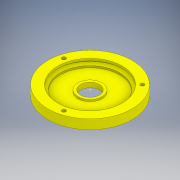
# Autodesk Inventor part: fix_plate_2
Saved by Autodesk Inventor 2018 (Build 220112000, 112)
## iProperties
Created: 2019-01-08
Part Number: fix_plate_2
Material: 一般
Document SubType Name: Modeling
Designer: lowyu
Density: 1 g/cm^3
Appearance: 既定
Author: lowyu
## iProperties of the stored document fix_plate_3D プリント.ipt
Created: 2019-01-08
Part Number: fix_plate_3D プリント
Material: 一般
Document SubType Name: Modeling
Designer: lowyu
Density: 1 g/cm^3
Appearance: 既定
Author: lowyu
Autodesk Inventor part; units mm, degrees
note: some values were not read from the file. Chosen so that the rebuilt part matches the saved one: second side of "押し出し6".
ref_plane "YZ Plane" through (0, 0, 0) normal (1, 0, 0) x (0, 1, 0)
ref_plane "XZ Plane" through (0, 0, 0) normal (0, 1, 0) x (-1, 0, 0)
ref_plane "XY Plane" through (0, 0, 0) normal (0, 0, 1) x (1, 0, 0)
sketch "スケッチ1" plane through (0, 0, 0) normal (0, 0, 1) x (1, 0, 0)
  circle A0 centre (0, 0) radius 46.9412
  dimension "d3" = 93.8824
  constraints: 1 centre point
  measures "d3" diameter of A0
extrude "押し出し1" add sketch "スケッチ1" along normal blind 10.5
sketch "スケッチ2" plane through (0, 0, 10.5) normal (0, 0, 1) x (1, 0, 0)
  circle A0 centre (0, 0) radius 46.9412
  arc A1 (35.7361, 3.8892) -> (3.8892, 35.7361) centre (0, 0) ccw
  circle A2 centre (29.2617, 29.2617) radius 2.1
  circle A3 centre (-39.9723, 10.7105) radius 2.1
  circle A4 centre (10.7105, -39.9723) radius 2.1
  circle A5 centre (0, 0) radius 35.9471
  dimension "d4" = 4.2
  constraints: 5 centre point, 2 point on circle, 1 coincident, 3 other
  measures "d4" diameter of A2
extrude "押し出し2" cut sketch "スケッチ2" against normal blind 5 contours A5 A1
sketch "スケッチ3" plane through (0, 0, 10.5) normal (0, 0, 1) x (1, 0, 0)
  circle A0 centre (0, 0) radius 46.9412
  arc A1 (-5.0225, 35.5945) -> (35.5945, -5.0225) centre (0, 0) ccw
  arc A2 (35.7361, 3.8892) -> (3.8892, 35.7361) centre (0, 0) ccw
  circle A3 centre (29.2617, 29.2617) radius 2.1
  circle A4 centre (-39.9723, 10.7105) radius 2.1
  circle A5 centre (10.7105, -39.9723) radius 2.1
  circle A6 centre (0, 0) radius 35.9471
  dimension "d7" = 4.2
  constraints: 6 centre point, 4 point on circle, 1 coincident, 3 other
  measures "d7" diameter of A3
extrude "押し出し3" cut sketch "スケッチ3" against normal blind 10.5 contours A3 | A4 | A5
sketch "スケッチ4" plane through (0, 0, 5.5) normal (0, 0, 1) x (1, 0, 0)
  circle A0 centre (0, 0) radius 10.5
  circle A1 centre (0, 0) radius 10.5
  constraints: 2 centre point
extrude "押し出し4" cut sketch "スケッチ4" against normal blind 10.5
sketch "スケッチ5" plane through (0, 0, 5.5) normal (0, 0, 1) x (1, 0, 0)
  circle A0 centre (0, 0) radius 10.5 projected
  circle A1 centre (0, 0) radius 35.9471 projected
  circle A2 centre (0, 0) radius 13.5
  circle A3 centre (0, 0) radius 32.9471
  dimension "d12" = 3
  dimension "d13" = 3
  constraints: 2 centre point, 2 coincident
  measures "d12" radial gap between concentric circles of A2 A0
  measures "d13" radial gap between concentric circles of A3 A1
extrude "押し出し5" cut sketch "スケッチ5" against normal blind 2 contours A3
sketch "スケッチ6" plane through (0, 0, 5.5) normal (0, 0, 1) x (1, 0, 0)
  point P0 (0, 0)
sketch "スケッチ7" plane through (0, 0, 5.5) normal (0, 0, 1) x (1, 0, 0)
  circle A0 centre (0, 0) radius 38.9471
  circle A1 centre (0, 0) radius 35.9471 projected
  dimension "d16" = 3
  constraints: 1 centre point, 1 coincident
  measures "d16" radial gap between concentric circles of A1 A0
extrude "押し出し6" cut sketch "スケッチ7" along normal blind 2.5
